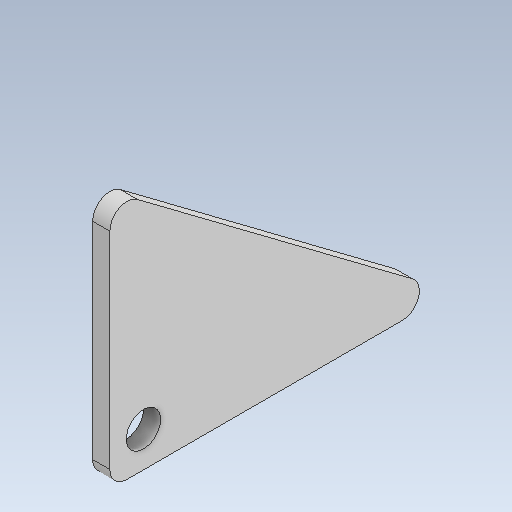
# Autodesk Inventor part: wing_horn
Saved by Autodesk Inventor 2021 (Build 250183000, 183)
## iProperties
Created: 2020-11-19
Part Number: wing_horn
Material: Generic
Document SubType Name: Modeling
Designer: Paco
Density: 1 g/cm^3
Appearance: Default
Mass: 0.144 g
Surface Area: 3.48566 cm^2
Volume: 0.144 cm^3
Author: Paco
Autodesk Inventor part; units mm, degrees
ref_plane "YZ Plane" through (0, 0, 0) normal (1, 0, 0) x (0, 1, 0)
ref_plane "XZ Plane" through (0, 0, 0) normal (0, 1, 0) x (-1, 0, 0)
ref_plane "XY Plane" through (0, 0, 0) normal (0, 0, 1) x (1, 0, 0)
sketch "Sketch1" plane through (0, 0, 0) normal (1, 0, 0) x (0, 1, 0)
  line L0 (6.712, 10.6489) -> (-8.288, 10.6489)
  line L1 (-8.288, 10.6489) -> (-8.288, -9.3511)
  line L2 (-8.288, -9.3511) -> (6.712, 10.6489)
  point P0 (0, 0)
  dimension "d0" = 20
  dimension "d1" = 15
  constraints: 6 end point, 1 horizontal, 1 perpendicular
  measures "d0" distance of L0.end L1.end
  measures "d1" distance of L0.start L0.end
extrude "Extrusion1" add sketch "Sketch1" along normal blind 1
fillet "Fillet1" radius 1 3 edges at (0.5, 6.712, 10.6489) (0.5, -8.288, 10.6489) (0.5, -8.288, -9.3511)
sketch "Sketch2" plane through (0, 0, 0) normal (-1, 0, 0) x (0, 0, 1)
  point P0 (0, 0)
  point P1 (8.6941, -6.2404)
hole "Hole1" at (0, -6.2404, 8.6941) direction (1, 0, 0) diameter 2 end through all
body "Solid1"
